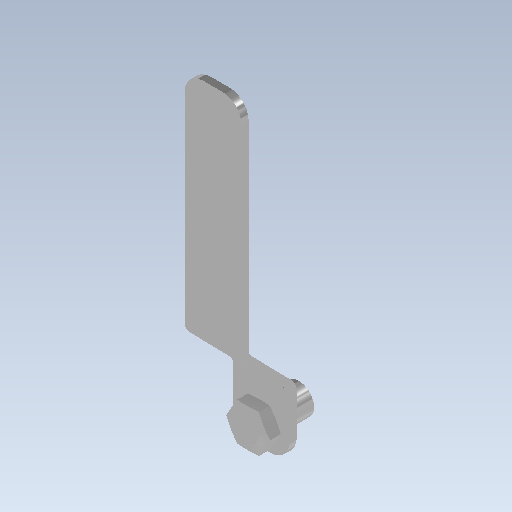
# Autodesk Inventor part: Flanged Ball Valve Handle
Saved by Autodesk Inventor 2020 (Build 240168000, 168)
## iProperties
Shininess: 41.0
Angle Display Precision: 2
Document Length Units: 11269
Document Angle Units: 11279
Document Time Units: 11290
Document Mass Units: 11283
Document Length Units Precision: 3
Document Angle Units Precision: 2
NAME: PIPING: BS4504 Flange PN16
DATA: <meta><inlinegroups number="0" deflen="0"></inlinegroups><connections number="1"></connections><angles></angles></meta>
Created: 2002-04-25
Part Number: Flanged Ball Valve Handle
Material: Cast Iron
Document SubType Name: Modeling
Designer: D.Ali
Description: Flanged Ball Valve Handle
Standard: BS4504
Standard Revision: 1
Manufacturer: Datech
Standards Organization: Custom
Language: ENG
Categories: <domain><piping version="1" type="fitting"><fitting><connection index="1" flipDirection="False"><display>Connection1</display><NS><bound-to>ND</bound-to></NS><Female>False</Female><EndTreatment>Flanged</EndTreatment><Fixed>False</Fixed><MaxEngagement> 0</MaxEngagement><MinEngagement> 0</MinEngagement></connection></fitting></piping></domain>
Density: 7.05 g/cm^3
Appearance: Metal-Steel (Polished)
Stock Number: NA
Mass: 189.855 g
Surface Area: 143.683 cm^2
Volume: 26.9299 cm^3
Density: 0.0
Volumn: 0.0
Area: 0.0
PropertySet Name: Model Information
Control State: 0
Master: False
Checked Out: False
Face_face: 229.000 mm
NB: 100.000 mm
PCD: 180.000 mm
FlangeOD: 220.000 mm
Holenum: 8.000 ul
FlangefaceOD: 156.000 mm
Holedia: 19.000 mm
Flangethk: 16.000 mm
PipeOD: 110.000 mm
Flangefacethk: 3.000 mm
Author: Demir Ali
Title: Purchased Part
Revision Number: A
Autodesk Inventor part; units mm, degrees
ref_plane "YZ Plane" through (0, 0, 0) normal (1, 0, 0) x (0, 1, 0)
ref_plane "Work Plane11" through (0, 89, 0) normal (0, -1, 0) x (1, 0, 0)
ref_plane "Work Plane12" through (0, 89, 62.5) normal (0, 0, 1) x (1, 0, 0)
sketch "Sketch60" plane through (0, 84.0068, 13.3927) normal (1, 0, 0) x (0, 0, -1)
  line L0 (-59.69, -7.4528) -> (-59.69, 24.2972)
  arc A0 (-59.69, 24.2972) -> (-61.8522, 29.6148) centre (-67.31, 24.2972) ccw
  line L1 (-61.8522, 29.6148) -> (-84.0089, 52.3556)
  arc A1 (-85.09, 55.0144) -> (-84.0089, 52.3556) centre (-81.28, 55.0144) ccw
  line L2 (-85.09, 55.0144) -> (-85.09, 170.3472)
  line L3 (-85.09, 170.3472) -> (-88.9, 170.3472)
  line L4 (-88.9, 170.3472) -> (-88.9, 55.0144)
  arc A2 (-88.9, 55.0144) -> (-86.7378, 49.6968) centre (-81.28, 55.0144) ccw
  line L5 (-86.7378, 49.6968) -> (-64.5811, 26.956)
  arc A3 (-63.5, 24.2972) -> (-64.5811, 26.956) centre (-67.31, 24.2972) ccw
  line L6 (-63.5, 24.2972) -> (-63.5, -7.4528)
  line L7 (-63.5, -7.4528) -> (-59.69, -7.4528)
  line L8 (0, -18.034) -> (0, 124.206)
  line L9 (-28.0662, 4.9932) -> (-56.6073, 4.9932)
  line L10 (-56.6073, -20.0068) -> (-56.6073, 29.9932)
  dimension "d306" = 3.81
  dimension "d307" = 3.81
  dimension "d308" = 3.81
  dimension "d304" = 177.8
  dimension "d311" = 31.75
  dimension "d309" = 31.75
  dimension "d305" = 25.4
  dimension "d310" = 59.69
  dimension "d303" = 12.446
  constraints: 22 end point, 8 point on circle, 8 tangent, 4 centre point, 4 vertical, 2 concentric, 2 horizontal, 1 midpoint, 1 parallel
  measures "d306" distance of L6.end L0.start
  measures "d307" radius of A3
  measures "d308" radius of A1
  measures "d304" distance between parallel lines of L3 L7
  measures "d311" distance of L0.start L0.end
  measures "d309" distance of L1.start L1.end
  measures "d305" distance between parallel lines of L4 L6
  measures "d310" distance between parallel lines of L8 L0
  measures "d303" distance between parallel lines of L7 L9
extrude "Extrusion43" add sketch "Sketch60" along normal mid plane 30
fillet "Fillet57" radius 10 4 edges at (-15, 76.554, 74.9877) (15, 76.554, 74.9877) (-15, 254.354, 100.3877) (15, 254.354, 100.3877)
sketch "Sketch61" plane through (-15, 108.304, 76.8927) normal (0, 0, 1) x (1, 0, 0)
  circle A0 centre (15, -19.304) radius 25
  circle A1 centre (15, -19.304) radius 8
  line L0 (3.453, -19.304) -> (9.2265, -9.304)
  line L1 (9.2265, -9.304) -> (20.7735, -9.304)
  line L2 (20.7735, -9.304) -> (26.547, -19.304)
  line L3 (26.547, -19.304) -> (20.7735, -29.304)
  line L4 (20.7735, -29.304) -> (9.2265, -29.304)
  line L5 (9.2265, -29.304) -> (3.453, -19.304)
  dimension "d321" = 16
  dimension "d324" = 20
  constraints: 12 end point, 2 centre point, 2 coincident, 11 other
  measures "d321" diameter of A1
  measures "d324" distance between parallel lines of L1 L4
extrude "Extrusion44" add sketch "Sketch61" against normal blind 20 contours A1
extrude "Extrusion45" add sketch "Sketch61" along normal blind 8 contours A1 | L0 L1 L2 L3 L4 L5
sketch "Sketch62" plane through (0, 0, 0) normal (1, 0, 0) x (0, 1, 0)
  line L0 (89, 76.8927) -> (79, 76.8927) projected
  line L1 (79, 84.8927) -> (89, 84.8927) projected
  line L2 (73.6393, 84.8927) -> (73.6393, 82.8927)
  line L3 (73.6393, 82.8927) -> (82.6108, 84.8927)
  line L4 (73.6393, 76.8927) -> (73.6393, 78.8927)
  line L5 (73.6393, 78.8927) -> (82.6108, 76.8927)
  line L6 (89, 115.9127) -> (89, 52.3527) projected
  line L7 (73.6393, 84.8927) -> (82.6108, 84.8927)
  line L8 (73.6393, 76.8927) -> (82.6108, 76.8927)
  dimension "d330" = 2
  constraints: 12 end point, 2 equal length, 2 perpendicular, 2 point on line, 2 vertical alignment, 1 collinear
  measures "d330" distance of L2.start L2.end
revolve "Revolution1" cut sketch "Sketch62" angle 360 about axis through (0, 89, 76.8927) along (0, 0, -1)
equation "\"NB\" = 50"
equation "\"PipeOD\" = 60.325"
equation "\"FlangeOD\" = 165"
equation "\"FlangefaceOD\" = 102"
equation "\"Holedia\" = 19"
equation "\"Holenum\" = 4"
equation "\"PCD\" = 125"
equation "\"Flangethk\" = 16"
equation "\"Flangefacethk\" = 3"
body "Solid1"
